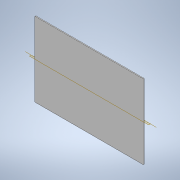
# Autodesk Inventor part: wire_half
Saved by Autodesk Inventor 2020 (Build 240168000, 168)
## iProperties
Created: 2021-01-20
Part Number: wire_half
Material: Generic
Document SubType Name: Modeling
Designer: phamv
Density: 1 g/cm^3
Appearance: Default
Author: phamv
Autodesk Inventor part; units mm, degrees
ref_plane "YZ Plane" through (0, 0, 0) normal (1, 0, 0) x (0, 1, 0)
ref_plane "XY Plane" through (0, 0, 0) normal (0, 0, 1) x (1, 0, 0)
sketch "Sketch1" plane through (0, 0, 0) normal (0, 0, 1) x (1, 0, 0)
  line L0 (0, -11.6) -> (500, -11.6)
  line L1 (500, -11.6) -> (500, -150)
  line L2 (500, -150) -> (-500, -150)
  line L3 (-500, -150) -> (-500, -38.8)
  line L4 (0, -11.6) -> (0, -15.6)
  line L5 (0, -15.6) -> (496, -15.6)
  line L6 (496, -15.6) -> (496, -146)
  line L7 (496, -146) -> (-496, -146)
  line L8 (-500, -38.8) -> (491, -38.8)
  line L9 (491, -38.8) -> (491, -141)
  line L10 (491, -141) -> (-491, -141)
  line L11 (-496, -146) -> (-496, -42.8)
  line L12 (-496, -42.8) -> (487, -42.8)
  line L13 (487, -42.8) -> (487, -137)
  line L14 (487, -137) -> (-487, -137)
  line L15 (-487, -137) -> (-487, -70)
  line L16 (-491, -141) -> (-491, -66)
  line L17 (-491, -66) -> (482, -66)
  line L18 (482, -66) -> (482, -132)
  line L19 (-487, -70) -> (478, -70)
  line L20 (478, -70) -> (478, -128)
  line L21 (-702, 0) -> (712, 0) projected
  line L22 (478, -128) -> (-482, -128)
  line L23 (482, -132) -> (-482, -132)
  line L24 (-482, -132) -> (-482, -128)
  line L25 (0, -150) -> (0, -11.6)
  point P0 (0, 0)
  point P1 (0, 0)
  dimension "d1" = 4
  dimension "d2" = 4
  dimension "d3" = 4
  dimension "d4" = 11.6
  dimension "d5" = 1000
  dimension "d6" = 500
  dimension "d7" = 4
  dimension "d8" = 4
  dimension "d9" = 5
  dimension "d10" = 4
  dimension "d11" = 23.2
  dimension "d12" = 4
  dimension "d13" = 5
  dimension "d14" = 4
  dimension "d15" = 4
  dimension "d16" = 4
  dimension "d17" = 5
  dimension "d19" = 23.2
  dimension "d20" = 5
  dimension "d82" = 150
  dimension "d88" = 4
  dimension "d89" = 5
  dimension "d90" = 5
  constraints: 50 end point, 15 perpendicular, 4 horizontal, 3 vertical, 2 parallel, 1 coincident, 1 collinear, 1 midpoint
  measures "d1" distance between parallel lines of L5 L0
  measures "d2" distance between parallel lines of L6 L1
  measures "d3" distance between parallel lines of L2 L7
  measures "d4" distance from line of L21 L0.start
  measures "d5" distance between parallel lines of L3 L1
  measures "d6" distance from line of point (0, 0) L1
  measures "d7" distance between parallel lines of L3 L11
  measures "d8" distance between parallel lines of L13 L9
  measures "d9" distance between parallel lines of L9 L6
  measures "d10" distance between parallel lines of L8 L12
  measures "d11" distance between parallel lines of L8 L5
  measures "d12" distance between parallel lines of L10 L14
  measures "d13" distance between parallel lines of L7 L10
  measures "d14" distance between parallel lines of L16 L15
  measures "d15" distance between parallel lines of L17 L19
  measures "d16" distance between parallel lines of L20 L18
  measures "d17" distance between parallel lines of L18 L13
  measures "d19" distance between parallel lines of L17 L12
  measures "d20" distance between parallel lines of L11 L16
  measures "d82" distance between parallel lines of L2 L21
  measures "d88" distance between parallel lines of L23 L22
  measures "d89" distance between parallel lines of L14 L23
  measures "d90" distance between parallel lines of L15 L24
extrude "Extrusion1" add sketch "Sketch1" along normal blind 4 contours L0 L1 L2 L25 L7 L6 L5 L4 | L25 L12 L11 L7 L2 L3 L8 | L8 L9 L10 L25 L14 L13 L12 | L25 L19 L15 L14 L10 L16 L17 | L17 L18 L23 L25 L22 L20 L19 | L25 L23 L24 L22
sketch "Sketch3" plane through (0, 0, 0) normal (0, 0, 1) x (1, 0, 0)
  line L0 (0, -15.6) -> (-500, -15.6)
  line L1 (-500, -15.6) -> (-500, 150)
  line L2 (-500, 150) -> (500, 150)
  line L3 (500, 150) -> (500, 11.6)
  line L4 (0, -11.6) -> (-496, -11.6)
  line L5 (-496, -11.6) -> (-496, 146)
  line L6 (-496, 146) -> (496, 146)
  line L7 (496, 146) -> (496, 15.6)
  line L8 (496, 15.6) -> (-487, 15.6)
  line L9 (-487, 15.6) -> (-487, 137)
  line L10 (500, 11.6) -> (-491, 11.6)
  line L11 (-491, 11.6) -> (-491, 141)
  line L12 (-487, 137) -> (487, 137)
  line L13 (-491, 141) -> (491, 141)
  line L14 (487, 137) -> (487, 42.8)
  line L15 (487, 42.8) -> (-478, 42.8)
  line L16 (491, 141) -> (491, 38.8)
  line L17 (491, 38.8) -> (-482, 38.8)
  line L18 (-478, 42.8) -> (-478, 128)
  line L19 (-478, 128) -> (479, 128)
  line L20 (479, 128) -> (479, 70)
  line L21 (479, 70) -> (-473, 70)
  line L22 (-482, 38.8) -> (-482, 132)
  line L23 (-482, 132) -> (483, 132)
  line L24 (483, 132) -> (483, 66)
  line L25 (483, 66) -> (-473, 66)
  line L26 (-473, 70) -> (-473, 66)
  line L27 (500, -150) -> (500, -11.6) projected
  line L28 (-702, 0) -> (712, 0) projected
  line L29 (0, 150) -> (0, -150) construction
  point P0 (0, 0)
  dimension "d58" = 4
  dimension "d59" = 4
  dimension "d60" = 4
  dimension "d61" = 5
  dimension "d62" = 5
  dimension "d64" = 4
  dimension "d65" = 4
  dimension "d66" = 4
  dimension "d67" = 5
  dimension "d68" = 1000
  dimension "d69" = 23.2
  dimension "d70" = 4
  dimension "d71" = 4
  dimension "d72" = 23.2
  dimension "d73" = 5
  dimension "d74" = 5
  dimension "d75" = 4
  dimension "d76" = 4
  dimension "d77" = 23.2
  dimension "d78" = 4
  dimension "d79" = 4
  dimension "d80" = 4
  dimension "d83" = 150
  dimension "d87" = 5
  constraints: 56 end point, 16 perpendicular, 4 parallel, 4 vertical, 3 horizontal, 1 collinear, 1 midpoint, 1 other
  measures "d58" distance between parallel lines of L1 L5
  measures "d59" distance between parallel lines of L2 L6
  measures "d60" distance between parallel lines of L7 L3
  measures "d61" distance between parallel lines of L13 L6
  measures "d62" distance between parallel lines of L5 L11
  measures "d64" distance between parallel lines of L10 L8
  measures "d65" distance between parallel lines of L14 L16
  measures "d66" distance between parallel lines of L13 L12
  measures "d67" distance between parallel lines of L16 L7
  measures "d68" distance between parallel lines of L1 L3
  measures "d69" distance between parallel lines of L4 L10
  measures "d70" distance between parallel lines of L11 L9
  measures "d71" distance between parallel lines of L17 L15
  measures "d72" distance between parallel lines of L8 L17
  measures "d73" distance between parallel lines of L12 L23
  measures "d74" distance between parallel lines of L9 L22
  measures "d75" distance between parallel lines of L23 L19
  measures "d76" distance between parallel lines of L24 L14
  measures "d77" distance between parallel lines of L15 L25
  measures "d78" distance between parallel lines of L24 L20
  measures "d79" distance between parallel lines of L25 L21
  measures "d80" distance between parallel lines of L22 L18
  measures "d83" distance of the line from the sketch origin of L2
  measures "d87" distance between parallel lines of L18 L26
extrude "Extrusion2" add sketch "Sketch3" along normal blind 4 fills toward (-248, -11.65) open curves L4 L5 L6 L7 L8 L9 L12 L14 L15 L18 L19 L20 L21 L26 L25 L24 L23 L22 L17 L16 L13 L11 L10 L3 L2 L1 L0
sketch "Sketch5" plane through (0, 0, 4) normal (0, 0, 1) x (1, 0, 0)
  line L0 (500, 150) -> (-500, 150) projected
  line L1 (-500, -150) -> (500, -150) projected
  line L2 (-500, 150) -> (0, 150)
  line L3 (0, 150) -> (0, -150)
  line L4 (0, -150) -> (-500, -150)
  line L5 (-500, -150) -> (-500, 150)
  point P0 (0, 0)
  constraints: 8 end point, 2 parallel, 1 horizontal, 1 midpoint, 1 perpendicular
extrude "Extrusion3" cut sketch "Sketch5" against normal up to surface (4 mm away)
sketch "Sketch6" plane through (0, 0, 4) normal (0, 0, 1) x (1, 0, 0)
  line L0 (0, 175) -> (510, 175)
  line L1 (510, 175) -> (510, -175)
  line L2 (510, -175) -> (0, -175)
  line L3 (0, -175) -> (0, 175)
  line L4 (500, 150) -> (0, 150) projected
  line L5 (0, -150) -> (500, -150) projected
  line L6 (500, 11.6) -> (500, 150) projected
  point P0 (0, 0)
  dimension "d93" = 25
  dimension "d94" = 25
  dimension "d95" = 10
  constraints: 8 end point, 2 parallel, 1 horizontal, 1 perpendicular
  measures "d93" distance between parallel lines of L4 L0
  measures "d94" distance between parallel lines of L2 L5
  measures "d95" distance between parallel lines of L1 L6
extrude "Extrusion4" add sketch "Sketch6" along normal blind 4
equation "\"d1\" = wire_diameter"
equation "\"d2\" = wire_diameter"
equation "\"d3\" = wire_diameter"
equation "\"d4\" = 0.5 * distance_between_wires"
equation "\"d5\" = track_length"
equation "\"d6\" = 0.5 * track_length"
equation "\"d7\" = wire_diameter"
equation "\"d8\" = wire_diameter"
equation "\"d9\" = distance_between_wires_edge"
equation "\"d10\" = wire_diameter"
equation "\"d11\" = distance_between_wires"
equation "\"d12\" = wire_diameter"
equation "\"d13\" = distance_between_wires_edge"
equation "\"d14\" = wire_diameter"
equation "\"d15\" = wire_diameter"
equation "\"d16\" = wire_diameter"
equation "\"d17\" = distance_between_wires_edge"
equation "\"d19\" = distance_between_wires"
equation "\"d20\" = distance_between_wires_edge"
equation "\"d82\" = 0.5 * track_width"
equation "\"d22\" = wire_diameter"
equation "\"d58\" = wire_diameter"
equation "\"d59\" = wire_diameter"
equation "\"d60\" = wire_diameter"
equation "\"d61\" = distance_between_wires_edge"
equation "\"d62\" = distance_between_wires_edge"
equation "\"d64\" = wire_diameter"
equation "\"d65\" = wire_diameter"
equation "\"d66\" = wire_diameter"
equation "\"d67\" = distance_between_wires_edge"
equation "\"d68\" = track_length"
equation "\"d69\" = distance_between_wires"
equation "\"d70\" = wire_diameter"
equation "\"d71\" = wire_diameter"
equation "\"d72\" = distance_between_wires"
equation "\"d73\" = distance_between_wires_edge"
equation "\"d74\" = distance_between_wires_edge"
equation "\"d75\" = wire_diameter"
equation "\"d76\" = wire_diameter"
equation "\"d77\" = distance_between_wires"
equation "\"d78\" = wire_diameter"
equation "\"d79\" = wire_diameter"
equation "\"d80\" = wire_diameter"
equation "\"d83\" = 0.5 * track_width"
equation "\"d85\" = wire_diameter"
equation "\"track_length\" = 1000"
equation "\"wire_diameter\" = 4"
equation "\"distance_between_wires\" = -1.2 * wire_diameter + 0.2 * parameter_6"
equation "\"distance_between_wires_edge\" = 5"
equation "\"d53\" = 5"
equation "\"d55\" = 5"
equation "\"d56\" = -1.2 * d53 + 0.2 * d57"
equation "\"d84\" = wire_diameter"
equation "\"track_width\" = 300"
equation "\"parameter_6\" = 140"
equation "\"d57\" = 120"
body "Solid1"
